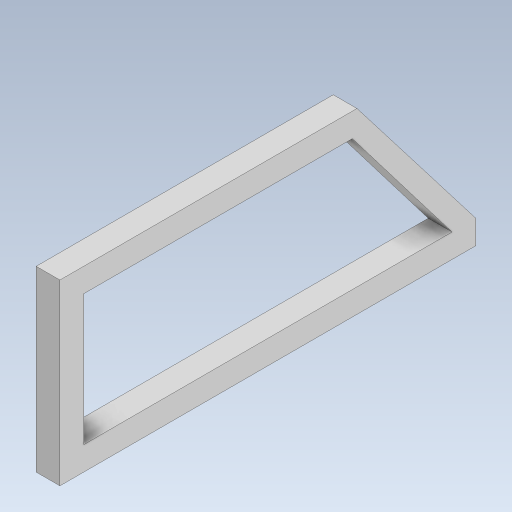
# Autodesk Inventor part: Holder Motor Lifter
Saved by Autodesk Inventor 2023.5 (Build 275446000, 446)
## iProperties
Created: 2025-09-06
Part Number: Holder Motor Lifter
Material: Generic
Document SubType Name: Modeling
Designer: Guntur
Density: 1 g/cm^3
Appearance: Default
Author: Guntur
## iProperties of the stored document Holder Motor Lifter_3DPrint.ipt
Created: 2025-09-06
Part Number: Holder Motor Lifter_3DPrint
Material: Generic
Document SubType Name: Modeling
Designer: Guntur
Density: 1 g/cm^3
Appearance: Default
Author: Guntur
Autodesk Inventor part; units mm, degrees
ref_plane "YZ Plane" through (0, 0, 0) normal (1, 0, 0) x (0, 1, 0)
ref_plane "XZ Plane" through (0, 0, 0) normal (0, 1, 0) x (-1, 0, 0)
ref_plane "XY Plane" through (0, 0, 0) normal (0, 0, 1) x (1, 0, 0)
sketch "Sketch1" plane through (0, 0, 0) normal (1, 0, 0) x (0, 1, 0)
  line L0 (0, 0) -> (-4, 0)
  line L1 (-4, 0) -> (-4, -70)
  line L2 (-4, -70) -> (0, -70)
  line L3 (0, -70) -> (0, -4)
  line L4 (-4, 0) -> (26, 0)
  line L5 (26, 0) -> (26, -4)
  line L6 (22, -4) -> (0, -4)
  line L7 (-4, -4) -> (-4, 0)
  line L8 (26, 0) -> (22, 0)
  line L9 (22, -4) -> (22, -50)
  line L10 (22, -50) -> (26, -50)
  line L11 (26, -50) -> (26, 0)
  line L12 (26, -50) -> (0, -70)
  line L13 (0, -70) -> (0, -66)
  line L14 (0, -66) -> (22, -49.2125)
  dimension "d0" = 4
  dimension "d1" = 70
  dimension "d2" = 30
  dimension "d3" = 4
  dimension "d4" = 4
  dimension "d5" = 50
  dimension "d6" = 4
  constraints: 30 end point, 6 parallel, 3 horizontal, 3 perpendicular, 2 point on line
  measures "d0" distance of L2.end L1.end
  measures "d1" distance of L1.end L0.end
  measures "d2" distance of L5.end L7.start
  measures "d3" distance of L4.end L5.end
  measures "d4" distance of L10.end L9.end
  measures "d5" distance of L9.end L8.end
  measures "d6" distance of L2.end L13.end
extrude "Extrusion1" add sketch "Sketch1" along normal blind 4 contours L4 L5 L11 L10 L9 L6 L3 L2 L1 L0 | L3 L14 L9 L10 L12
body "Solid1"
